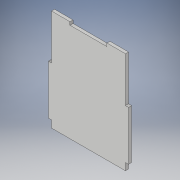
# Autodesk Inventor part: front
Saved by Autodesk Inventor 2019 (Build 230136000, 136)
## iProperties
Created: 2018-09-07
Part Number: front
Material: Generic
Document SubType Name: Modeling
Designer: mspet
Density: 1 g/cm^3
Appearance: Default
Author: mspet
Autodesk Inventor part; units mm, degrees
ref_plane "YZ Plane" through (0, 0, 0) normal (1, 0, 0) x (0, 1, 0)
ref_plane "XZ Plane" through (0, 0, 0) normal (0, 1, 0) x (-1, 0, 0)
ref_plane "XY Plane" through (0, 0, 0) normal (0, 0, 1) x (1, 0, 0)
sketch "Sketch1" plane through (0, 0, 0) normal (0, 0, 1) x (1, 0, 0)
  line L0 (0, 0) -> (76.2, 0)
  line L1 (76.2, 0) -> (76.2, 79.0194)
  line L2 (76.2, 79.0194) -> (0, 79.0194)
  line L3 (0, 79.0194) -> (0, 0)
  line L4 (0, 7.3406) -> (-3.175, 7.3406)
  line L5 (-3.175, 7.3406) -> (-3.175, 58.1406)
  line L6 (-3.175, 58.1406) -> (0, 58.1406)
  line L7 (0, 58.1406) -> (0, 7.3406)
  line L8 (38.1, 79.0194) -> (38.1, 15.1376) construction
  line L9 (76.2, 0) -> (0, 0)
  line L10 (76.2, 79.0194) -> (76.2, 0)
  line L11 (76.2, 7.3406) -> (79.375, 7.3406)
  line L12 (79.375, 7.3406) -> (79.375, 58.1406)
  line L13 (79.375, 58.1406) -> (76.2, 58.1406)
  line L14 (76.2, 58.1406) -> (76.2, 7.3406)
  dimension "d0" = 76.2
  dimension "d1" = 79.0194
  dimension "d2" = 7.3406
  dimension "d3" = 50.8
  dimension "d6" = 3.175
  constraints: 30 end point, 6 symmetric about line, 4 parallel, 2 horizontal, 2 perpendicular, 2 point on line, 1 midpoint, 1 vertical
  measures "d0" distance of L1.end L2.end
  measures "d1" distance of L0.end L1.end
  measures "d2" distance between parallel lines of L4 L0
  measures "d3" distance of L4.end L5.end
  measures "d6" distance of L5.end L6.end
extrude "Extrusion1" add sketch "Sketch1" along normal blind 3.175
sketch "Sketch2" plane through (0, 0, 3.175) normal (0, 0, 1) x (1, 0, 0)
  line L0 (76.2, 79.0194) -> (0, 79.0194) projected
  line L1 (0, 79.0194) -> (76.2, 79.0194)
  line L2 (76.2, 79.0194) -> (76.2, 104.4194)
  line L3 (76.2, 104.4194) -> (0, 104.4194)
  line L4 (0, 104.4194) -> (0, 79.0194)
  point P0 (0, 0)
  dimension "d7" = 25.4
  constraints: 8 end point, 2 parallel, 1 horizontal, 1 perpendicular
  measures "d7" distance of L1.end L2.end
extrude "Extrusion2" add sketch "Sketch2" against normal blind 3.175
sketch "Sketch3" plane through (0, 0, 3.175) normal (0, 0, 1) x (1, 0, 0)
  line L0 (76.2, 104.4194) -> (0, 104.4194) projected
  line L1 (19.05, 104.4194) -> (57.15, 104.4194)
  line L2 (57.15, 104.4194) -> (57.15, 101.2444)
  line L3 (57.15, 101.2444) -> (19.05, 101.2444)
  line L4 (19.05, 101.2444) -> (19.05, 104.4194)
  line L5 (0, 104.4194) -> (0, 58.1406) projected
  point P0 (0, 0)
  dimension "d10" = 3.175
  dimension "d11" = 38.1
  dimension "d12" = 19.05
  constraints: 8 end point, 2 parallel, 1 horizontal, 1 perpendicular, 1 point on line
  measures "d10" distance of L1.end L2.end
  measures "d11" distance of L2.end L3.end
  measures "d12" distance between parallel lines of L5 L4
extrude "Extrusion3" cut sketch "Sketch3" against normal blind 3.175
body "Solid1"
